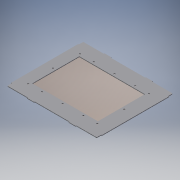
# Autodesk Inventor part: BrennerHalter
Saved by Autodesk Inventor 2018 (Build 220112000, 112)
## iProperties
Created: 2017-11-12
Part Number: BrennerHalter
Material: Generisch
Document SubType Name: Blech
Density: 1 g/cm^3
Sheet Metal Rule: Standard_mm
Appearance: Vorgabe
Flat Pattern Width: 26.29 cm
Flat Pattern Length: 22.39 cm
Flat Pattern Area: 588.633 cm^2
Sheet Metal Width: 262,900 mm
Sheet Metal Length: 223,900 mm
Sheet Metal Area: 58863,266 mm^2
Autodesk Inventor part; units mm, degrees
ref_plane "YZ Plane" through (0, 0, 0) normal (1, 0, 0) x (0, 1, 0)
ref_plane "XZ Plane" through (0, 0, 0) normal (0, 1, 0) x (-1, 0, 0)
ref_plane "XY Plane" through (0, 0, 0) normal (0, 0, 1) x (1, 0, 0)
ref_plane "Arbeitsebene1" through (0, 0, 0) normal (0, 0, 1) x (1, 0, 0)
sketch "Skizze1" plane through (0, 0, 0) normal (0, 0, 1) x (1, 0, 0)
  line L0 (53.9, 111.9999) -> (53.9, 109.9999) construction
  line L1 (53.9, 109.9999) -> (-45.9, 109.9999) construction
  line L2 (-45.9, 109.9999) -> (-45.9, 111.9999) construction
  line L3 (-66.1, 111.9999) -> (-66.1, 109.9999) construction
  line L4 (-66.1, 109.9999) -> (-123.5, 109.9999) construction
  arc A0 (-123.5, 109.9999) -> (-125.5, 107.9999) centre (-123.5, 107.9999) ccw construction
  line L5 (-125.5, 107.9999) -> (-125.5, 96.9999) construction
  line L6 (-125.5, 96.9999) -> (-127.5, 96.9999) construction
  line L7 (133.5, 96.9999) -> (133.5, 107.9999) construction
  arc A1 (133.5, 107.9999) -> (131.5, 109.9999) centre (131.5, 107.9999) ccw construction
  line L8 (131.5, 109.9999) -> (74.1, 109.9999) construction
  line L9 (74.1, 109.9999) -> (74.1, 111.9999) construction
  line L10 (135.5, 96.9999) -> (133.5, 96.9999) construction
  line L11 (-45.9, -111.9999) -> (-45.9, -109.9999) construction
  line L12 (-45.9, -109.9999) -> (53.9, -109.9999) construction
  line L13 (53.9, -109.9999) -> (53.9, -111.9999) construction
  line L14 (74.1, -111.9999) -> (74.1, -109.9999) construction
  line L15 (74.1, -109.9999) -> (131.5, -109.9999) construction
  arc A2 (131.5, -109.9999) -> (133.5, -107.9999) centre (131.5, -107.9999) ccw construction
  line L16 (133.5, -107.9999) -> (133.5, -96.9999) construction
  line L17 (133.5, -96.9999) -> (135.5, -96.9999) construction
  line L18 (-125.5, -96.9999) -> (-125.5, -107.9999) construction
  arc A3 (-125.5, -107.9999) -> (-123.5, -109.9999) centre (-123.5, -107.9999) ccw construction
  line L19 (-123.5, -109.9999) -> (-66.1, -109.9999) construction
  line L20 (-66.1, -109.9999) -> (-66.1, -111.9999) construction
  line L21 (-127.5, -96.9999) -> (-125.5, -96.9999) construction
  line L22 (135.5, -96.9999) -> (135.5, 96.9999) construction
  line L23 (74.1, 111.9999) -> (53.9, 111.9999) construction
  line L24 (-45.9, 111.9999) -> (-66.1, 111.9999) construction
  line L25 (-127.5, 96.9999) -> (-127.5, -96.9999) construction
  line L26 (-127.5, -109.9999) -> (-127.5, -111.9999) construction
  line L27 (-66.1, -111.9999) -> (-45.9, -111.9999) construction
  line L28 (53.9, -111.9999) -> (74.1, -111.9999) construction
  line L29 (135.45, 96.9499) -> (133.45, 96.9499)
  line L30 (133.45, 96.9499) -> (133.45, 107.9999)
  arc A4 (133.45, 107.9999) -> (131.5, 109.9499) centre (131.5, 107.9999) ccw
  line L31 (131.5, 109.9499) -> (74.05, 109.9499)
  line L32 (74.05, 109.9499) -> (74.05, 111.9499)
  line L33 (74.05, 111.9499) -> (53.95, 111.9499)
  line L34 (53.95, 111.9499) -> (53.95, 109.9499)
  line L35 (53.95, 109.9499) -> (-45.95, 109.9499)
  line L36 (-45.95, 109.9499) -> (-45.95, 111.9499)
  line L37 (-45.95, 111.9499) -> (-66.05, 111.9499)
  line L38 (-66.05, 111.9499) -> (-66.05, 109.9499)
  line L39 (-66.05, 109.9499) -> (-123.5, 109.9499)
  arc A5 (-123.5, 109.9499) -> (-125.45, 107.9999) centre (-123.5, 107.9999) ccw
  line L40 (-125.45, 107.9999) -> (-125.45, 96.9499)
  line L41 (-125.45, 96.9499) -> (-127.45, 96.9499)
  line L42 (-127.45, 96.9499) -> (-127.45, -96.9499)
  line L43 (-127.45, -96.9499) -> (-125.45, -96.9499)
  line L44 (-125.45, -96.9499) -> (-125.45, -107.9999)
  arc A6 (-125.45, -107.9999) -> (-123.5, -109.9499) centre (-123.5, -107.9999) ccw
  line L45 (-123.5, -109.9499) -> (-66.05, -109.9499)
  line L46 (-66.05, -109.9499) -> (-66.05, -111.9499)
  line L47 (-66.05, -111.9499) -> (-45.95, -111.9499)
  line L48 (-45.95, -111.9499) -> (-45.95, -109.9499)
  line L49 (-45.95, -109.9499) -> (53.95, -109.9499)
  line L50 (53.95, -109.9499) -> (53.95, -111.9499)
  line L51 (53.95, -111.9499) -> (74.05, -111.9499)
  line L52 (74.05, -111.9499) -> (74.05, -109.9499)
  line L53 (74.05, -109.9499) -> (131.5, -109.9499)
  arc A7 (131.5, -109.9499) -> (133.45, -107.9999) centre (131.5, -107.9999) ccw
  line L54 (133.45, -107.9999) -> (133.45, -96.9499)
  line L55 (133.45, -96.9499) -> (135.45, -96.9499)
  line L56 (135.45, -96.9499) -> (135.45, 96.9499)
  circle A8 centre (99.9961, 75.0051) radius 2.25
  circle A9 centre (59.9961, 75.0041) radius 2.25
  circle A10 centre (102.9981, 0.0052) radius 2.25
  circle A11 centre (100, -74.9949) radius 2.25
  circle A12 centre (60, -74.9959) radius 2.25
  circle A13 centre (0, -74.9974) radius 2.25
  circle A14 centre (-60, -74.999) radius 2.25
  circle A15 centre (-100, -75) radius 2.25
  circle A16 centre (-100.0039, 75) radius 2.25
  circle A17 centre (-60.0039, 75.001) radius 2.25
  circle A18 centre (-0.0039, 75.0026) radius 2.25
  line L57 (100, -74.9949) -> (-100.0039, 75) construction
  line L58 (-100.0039, 75) -> (99.9961, 75.0051) construction
  line L59 (99.9961, 75.0051) -> (-100, -75) construction
  line L60 (94.9981, 68.0026) -> (-95.0019, 68.0026)
  line L61 (-95.0019, 68.0026) -> (-95.0019, -67.9974)
  line L62 (-95.0019, -67.9974) -> (94.9981, -67.9974)
  line L63 (94.9981, -67.9974) -> (94.9981, 68.0026)
  line L64 (94.9981, 68.0026) -> (-95.0019, -67.9974) construction
  line L65 (-95.0019, 68.0026) -> (94.9981, -67.9974) construction
  circle A19 centre (-103.0019, -0.0001) radius 2.25
  point P0 (0, 0)
  point P1 (-0.0019, 0.0026)
  dimension "d0" = 0.05
  dimension "d1" = 190
  dimension "d2" = 136
  measures "d0" distance between parallel lines of L22 L56
  measures "d1" distance of L62.end L61.end
  measures "d2" distance of L61.end L60.end
extrude "Grobblech1" add sketch "Skizze1" along normal blind 2
equation "\"d3\" = Stärke"
equation "\"Biegeradius\" = Stärke"
equation "\"BreiteBiegungsfreistellung\" = Stärke"
equation "\"TiefeBiegungsfreistellung\" = 0.5 * Stärke"
equation "\"GrößeEckenfreistellung\" = 4 * Stärke"
equation "\"MinimalRest\" = 2 * Stärke"
equation "\"Übergangsradius\" = Biegeradius"
equation "\"JacobiRadiusGröße\" = Biegeradius"
equation "\"Abstandsgröße\" = Stärke"
equation "\"Stärke\" = 2"
